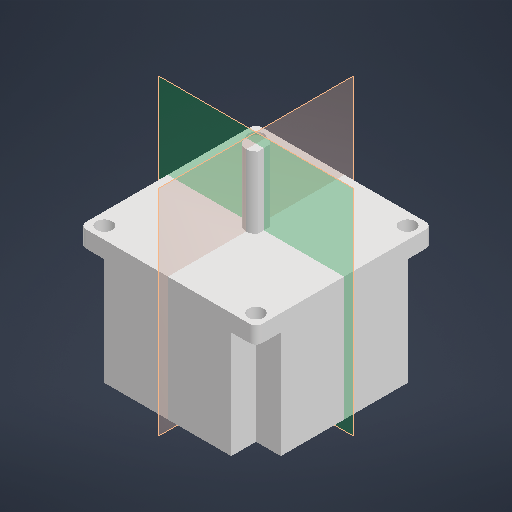
# Autodesk Inventor part: Motor
Saved by Autodesk Inventor 2026.1 (Build 301233020, 233B)
## iProperties
Created: 2025-12-03
Part Number: Motor
Material: Generic
Document SubType Name: Modeling
Designer: Mikke
Density: 1 g/cm^3
Appearance: Default
Author: Mikke
Autodesk Inventor part; units mm, degrees
ref_plane "YZ Plane" through (0, 0, 0) normal (1, 0, 0) x (0, 1, 0)
ref_plane "XZ Plane" through (0, 0, 0) normal (0, 1, 0) x (-1, 0, 0)
ref_plane "XY Plane" through (0, 0, 0) normal (0, 0, 1) x (1, 0, 0)
sketch "Sketch1" plane through (0, 0, 0) normal (0, 1, 0) x (-1, 0, 0)
  line L0 (-28.5, 28.5) -> (28.5, 28.5)
  line L1 (28.5, 28.5) -> (28.5, -28.5)
  line L2 (28.5, -28.5) -> (-28.5, -28.5)
  line L3 (-28.5, -28.5) -> (-28.5, 28.5)
  line L4 (-28.5, 28.5) -> (28.5, -28.5) construction
  line L5 (28.5, 28.5) -> (-28.5, -28.5) construction
  line L6 (28.5, -28.5) -> (20.5, -28.5)
  line L7 (20.5, -28.5) -> (20.5, -20.5)
  line L8 (20.5, -20.5) -> (28.5, -20.5)
  line L9 (28.5, -20.5) -> (28.5, -28.5)
  line L10 (-28.5, -28.5) -> (-22.5, -28.5)
  line L11 (-22.5, -28.5) -> (-22.5, -20.5)
  line L12 (-22.5, -20.5) -> (-28.5, -20.5)
  line L13 (-28.5, -20.5) -> (-28.5, -28.5)
  line L14 (-28.5, 28.5) -> (-20.5, 28.5)
  line L15 (-20.5, 28.5) -> (-20.5, 20.5)
  line L16 (-20.5, 20.5) -> (-28.5, 20.5)
  line L17 (-28.5, 20.5) -> (-28.5, 28.5)
  line L18 (28.5, 28.5) -> (20.5, 28.5)
  line L19 (20.5, 28.5) -> (20.5, 20.5)
  line L20 (20.5, 20.5) -> (28.5, 20.5)
  line L21 (28.5, 20.5) -> (28.5, 28.5)
  line L22 (-28.5, -28.5) -> (-20.5, -28.5)
  line L23 (-20.5, -28.5) -> (-20.5, -20.5)
  line L24 (-20.5, -20.5) -> (-28.5, -20.5)
  line L25 (-28.5, -20.5) -> (-28.5, -28.5)
  point P0 (0, 0)
  point P1 (28.5, 20.5)
  point P2 (20.5, 28.5)
  point P3 (-20.5, 28.5)
  point P4 (-28.5, 20.5)
  point P5 (-28.5, -20.5)
  point P6 (20.5, -28.5)
  dimension "d0" = 57
  dimension "d1" = 57
  dimension "d2" = 8
  dimension "d3" = 8
  dimension "d4" = 6
  dimension "d5" = 8
  dimension "d6" = 8
  dimension "d7" = 8
  dimension "d8" = 8
  dimension "d9" = 8
  dimension "d19" = 8
  dimension "d20" = 8
  constraints: 52 end point, 12 parallel, 6 horizontal, 6 perpendicular, 2 midpoint, 1 point on line
  measures "d0" distance of L1.end L2.end
  measures "d1" distance of L0.end L1.end
  measures "d2" distance of L7.end L8.end
  measures "d3" distance of L6.end L7.end
  measures "d4" distance of L12.end L11.end
  measures "d5" distance of L11.end L10.end
  measures "d6" distance of L15.end L16.end
  measures "d7" distance of L14.end L15.end
  measures "d8" distance of L20.end L19.end
  measures "d9" distance of L19.end L18.end
  measures "d19" distance of L24.end L23.end
  measures "d20" distance of L23.end L22.end
extrude "Extrusion1" add sketch "Sketch1" along normal blind 40 contours L0 L19 L20 L1 L8 L7 L2 L23 L24 L12 L3 L16 L15
sketch "Sketch2" plane through (0, 40, 0) normal (0, 1, 0) x (1, 0, 0)
  line L0 (-20.5, -20.5) -> (-20.5, -28.5) projected
  line L1 (-20.5, -28.5) -> (20.5, -28.5) projected
  line L2 (20.5, -28.5) -> (20.5, -20.5) projected
  line L3 (20.5, -20.5) -> (28.5, -20.5) projected
  line L4 (28.5, -20.5) -> (28.5, 20.5) projected
  line L5 (28.5, 20.5) -> (20.5, 20.5) projected
  line L6 (20.5, 28.5) -> (-20.5, 28.5) projected
  line L7 (-20.5, 28.5) -> (-20.5, 20.5) projected
  line L8 (-20.5, 20.5) -> (-28.5, 20.5) projected
  line L9 (-28.5, 20.5) -> (-28.5, -20.5) projected
  line L10 (-28.5, -20.5) -> (-20.5, -20.5) projected
  circle A0 centre (0, 0) radius 3.25
  line L11 (20.5, 20.5) -> (20.5, 28.5) projected
  line L12 (-3.25, 0) -> (2.55, 0)
  line L13 (2.55, 2.0149) -> (2.55, -2.0149)
  dimension "d12" = 6.5
  dimension "d24" = 5.8
  constraints: 4 end point, 2 point on circle, 1 centre point, 1 coincident, 1 horizontal, 1 midpoint, 1 vertical
  measures "d12" diameter of A0
  measures "d24" distance of L12.start L12.end
extrude "Extrusion2" add sketch "Sketch2" along normal blind 23 contours L13 L12 A0 | A0 L12 L13
sketch "Sketch3" plane through (0, 40, 0) normal (0, 1, 0) x (1, 0, 0)
  arc A0 (2.55, 2.0149) -> (2.55, -2.0149) centre (0, 0) ccw projected
  line L0 (-20.5, -20.5) -> (-20.5, -28.5) projected
  line L1 (-20.5, -28.5) -> (20.5, -28.5) projected
  line L2 (20.5, -28.5) -> (20.5, -20.5) projected
  line L3 (20.5, -20.5) -> (28.5, -20.5) projected
  line L4 (28.5, -20.5) -> (28.5, 20.5) projected
  line L5 (28.5, 20.5) -> (20.5, 20.5) projected
  line L6 (20.5, 28.5) -> (-20.5, 28.5) projected
  line L7 (-20.5, 28.5) -> (-20.5, 20.5) projected
  line L8 (-20.5, 20.5) -> (-28.5, 20.5) projected
  line L9 (-28.5, 20.5) -> (-28.5, -20.5) projected
  line L10 (-28.5, -20.5) -> (-20.5, -20.5) projected
  line L11 (-28.5, -28.5) -> (28.5, -28.5)
  line L12 (28.5, -28.5) -> (28.5, 28.5)
  line L13 (28.5, 28.5) -> (-28.5, 28.5)
  line L14 (-28.5, 28.5) -> (-28.5, -28.5)
  line L15 (20.5, 20.5) -> (20.5, 28.5) projected
  line L16 (2.55, 2.0149) -> (2.55, -2.0149) projected
  point P0 (-28.5, 20.5)
  point P1 (-28.5, -20.5)
  point P2 (-20.5, -28.5)
  point P3 (20.5, -28.5)
  point P4 (28.5, -20.5)
  point P5 (28.5, 20.5)
  constraints: 8 end point, 2 parallel, 1 horizontal, 1 perpendicular
extrude "Extrusion3" add sketch "Sketch3" against normal blind 5.4 contours L16 A0 | L10 L9 L8 L7 L6 L15 L5 L4 L3 L2 L1 L0 | L0 L11 L14 L10 | L2 L3 L12 L11 | L14 L13 L7 L8 | L5 L15 L13 L12
fillet "Fillet1" radius 2 4 edges at (28.5, 37.3, 28.5) (-28.5, 37.3, 28.5) (-28.5, 37.3, -28.5) (28.5, 37.3, -28.5)
sketch "Sketch4" plane through (0, 40, 0) normal (0, 1, 0) x (1, 0, 0)
  line L0 (-20.5, 20.5) -> (-28.5, 20.5) projected
  line L1 (-20.5, 28.5) -> (-20.5, 20.5) projected
  line L2 (20.5, 28.5) -> (-20.5, 28.5) projected
  line L3 (28.5, 20.5) -> (20.5, 20.5) projected
  line L4 (28.5, -20.5) -> (28.5, 20.5) projected
  line L5 (20.5, -20.5) -> (28.5, -20.5) projected
  line L6 (20.5, -28.5) -> (20.5, -20.5) projected
  line L7 (-20.5, -28.5) -> (20.5, -28.5) projected
  line L8 (-20.5, -20.5) -> (-20.5, -28.5) projected
  line L9 (-28.5, -20.5) -> (-20.5, -20.5) projected
  line L10 (-28.5, 20.5) -> (-28.5, -20.5) projected
  line L11 (20.5, -20.5) -> (28.5, -20.5) projected
  line L12 (20.5, -20.5) -> (28.5, -20.5)
  line L13 (28.5, -20.5) -> (28.5, -28.5)
  line L14 (28.5, -28.5) -> (20.5, -28.5)
  line L15 (20.5, -28.5) -> (20.5, -20.5)
  line L16 (20.5, 20.5) -> (20.5, 28.5) projected
  circle A0 centre (24.5, -24.5) radius 2.5
  point P0 (0, 0)
  dimension "d21" = 5
  constraints: 8 end point, 2 parallel, 1 centre point, 1 horizontal, 1 perpendicular
  measures "d21" diameter of A0
extrude "Extrusion4" cut sketch "Sketch4" against normal blind 40 contours A0
ref_plane "Work Plane1" through (0, 0, 20.5) normal (1, 0, 0) x (0, 0, -1)
ref_plane "Work Plane2" through (20.5, 0, 0) normal (0, 0, -1) x (-1, 0, 0)
mirror "Mirror1" about plane through (0, 0, 20.5) normal (1, 0, 0) of "Extrusion4"
mirror "Mirror2" about plane through (20.5, 0, 0) normal (0, 0, -1) of "Extrusion4", "Mirror1"
body "Solid1"
